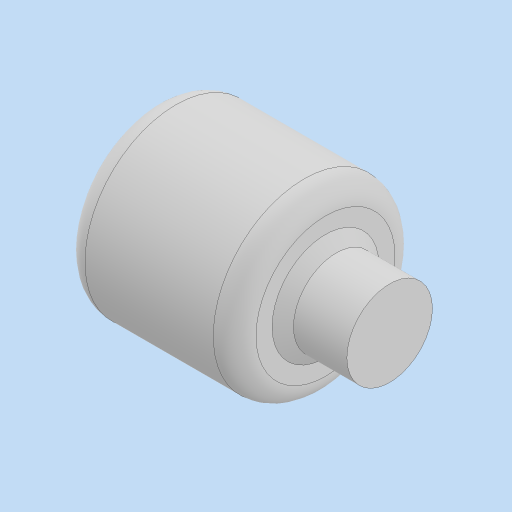
# Autodesk Inventor part: scroll_wheel
Saved by Autodesk Inventor 2024 (Build 280153000, 153)
## iProperties
Created: 2025-05-08
Part Number: scroll_wheel
Material: Generic
Document SubType Name: Modeling
Designer: XxPan
Density: 1 g/cm^3
Appearance: Default
Author: XxPan
Autodesk Inventor part; units mm, degrees
ref_plane "YZ Plane" through (0, 0, 0) normal (1, 0, 0) x (0, 1, 0)
ref_plane "XZ Plane" through (0, 0, 0) normal (0, 1, 0) x (-1, 0, 0)
ref_plane "XY Plane" through (0, 0, 0) normal (0, 0, 1) x (1, 0, 0)
sketch "Sketch1" plane through (0, 0, 0) normal (1, 0, 0) x (0, 1, 0)
  circle A0 centre (0, 0) radius 8.5
  dimension "d0" = 17
  constraints: 1 centre point, 1 coincident
  measures "d0" diameter of A0
extrude "Extrusion1" add sketch "Sketch1" along normal mid plane 16
sketch "Sketch2" plane through (8, 0, 0) normal (1, 0, 0) x (0, 0, -1)
  circle A0 centre (0, 0) radius 4
  dimension "d3" = 8
  constraints: 1 centre point, 1 coincident
  measures "d3" diameter of A0
extrude "Extrusion2" add sketch "Sketch2" along normal blind 6
sketch "Sketch3" plane through (-8, 0, 0) normal (-1, 0, 0) x (0, 0, 1)
  circle A0 centre (0, 0) radius 4 projected
  line L0 (0.4619, 0.8) -> (0.9238, 0)
  line L1 (0.9238, 0) -> (0.4619, -0.8)
  line L2 (0.4619, -0.8) -> (-0.4619, -0.8)
  line L3 (-0.4619, -0.8) -> (-0.9238, 0)
  line L4 (-0.9238, 0) -> (-0.4619, 0.8)
  line L5 (-0.4619, 0.8) -> (0.4619, 0.8)
  dimension "d6" = 1.6
  constraints: 12 end point, 1 coincident, 13 other
  measures "d6" distance between parallel lines of L2 L5
extrude "Extrusion3" add sketch "Sketch3" along normal blind 3 contours L0 L1 L2 L3 L4 L5
chamfer "Chamfer1" distance 1 angle 45 1 edges at (8, 0, 4)
fillet "Fillet1" radius 2 2 edges at (8, -8.5, 0) (-8, -8.5, 0)
fillet "Fillet2" radius 1 6 edges at (-8, 0.8, 0) (-8, 0.4, 0.6928) (-8, -0.4, 0.6928) (-8, -0.8, 0) (-8, 0.4, -0.6928) (-8, -0.4, -0.6928)
equation "\"BendRadius\" = Thickness"
equation "\"BendReliefWidth\" = Thickness"
equation "\"BendReliefDepth\" = 0.5 * Thickness"
equation "\"CornerReliefSize\" = 4 * Thickness"
equation "\"MinimumRemnant\" = 2 * Thickness"
equation "\"TransitionRadius\" = BendRadius"
equation "\"JacobiRadiusSize\" = BendRadius"
equation "\"GapSize\" = Thickness"
equation "\"Thickness\" = 3.048"
body "Solid1"
